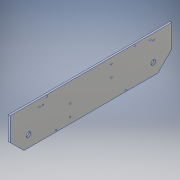
# Autodesk Inventor part: DriveTrain3.0
Saved by Autodesk Inventor 2019 (Build 230136000, 136)
## iProperties
Created: 2017-07-22
Part Number: DriveTrain3.0
Material: Aluminum 6061
Document SubType Name: Modeling
Designer: User
Density: 2.7 g/cm^3
Appearance: Aluminum - Flat
Mass: 590.045 g
Surface Area: 982.684 cm^2
Volume: 218.535 cm^3
Author: User
Autodesk Inventor part; units mm, degrees
ref_plane "YZ Plane" through (0, 0, 0) normal (1, 0, 0) x (0, 1, 0)
ref_plane "XZ Plane" through (0, 0, 0) normal (0, 1, 0) x (-1, 0, 0)
ref_plane "XY Plane" through (0, 0, 0) normal (0, 0, 1) x (1, 0, 0)
sketch "Sketch1" plane through (0, 0, 0) normal (1, 0, 0) x (0, 1, 0)
  line L0 (0, 0) -> (101.6, 0)
  line L1 (101.6, 0) -> (101.6, -444.5)
  line L2 (101.6, -444.5) -> (0, -444.5)
  line L3 (0, -444.5) -> (0, 0)
  circle A0 centre (31.75, -50.8) radius 6.3627
  circle A1 centre (31.75, -393.7) radius 6.3627
  circle A2 centre (86.2838, -165.5318) radius 1.5875
  circle A3 centre (70.2818, -165.5318) radius 1.5875
  circle A4 centre (15.3162, -278.9682) radius 1.5875
  circle A5 centre (31.3182, -278.9682) radius 1.5875
  dimension "d0" = 101.6
  dimension "d1" = 444.5
  dimension "d2" = 12.7254
  dimension "d3" = 31.75
  dimension "d4" = 50.8
  dimension "d5" = 50.8
  dimension "d22" = 165.5318
  dimension "d23" = 3.175
  dimension "d24" = 15.3162
  dimension "d25" = 3.175
  dimension "d26" = 16.002
  dimension "d27" = 165.5318
  dimension "d28" = 3.175
  dimension "d29" = 15.3162
  dimension "d30" = 165.5318
  dimension "d31" = 3.175
  dimension "d32" = 16.002
  dimension "d33" = 165.5318
  constraints: 8 end point, 6 centre point, 2 parallel, 1 horizontal, 1 perpendicular
  measures "d0" distance of L1.end L2.end
  measures "d1" distance of L0.end L1.end
  measures "d2" diameter of A0
  measures "d3" distance from line of L3 A0.centre
  measures "d4" distance from line of L0 A0.centre
  measures "d5" distance from line of L2 A1.centre
  measures "d22" distance from line of L0 A2.centre
  measures "d23" diameter of A2
  measures "d24" distance from line of L1 A2.centre
  measures "d25" diameter of A3
  measures "d26" distance of A2.centre A3.centre
  measures "d27" distance from line of L0 A3.centre
  measures "d28" diameter of A4
  measures "d29" distance from line of L3 A4.centre
  measures "d30" distance from line of L2 A4.centre
  measures "d31" diameter of A5
  measures "d32" distance of A5.centre A4.centre
  measures "d33" distance from line of L2 A5.centre
extrude "Extrusion1" add sketch "Sketch1" along normal blind 4.7625 contours L0 L1 L2 L3 | A2 | A3 | A4 | A5
chamfer "Chamfer1" distance 38.1 angle 45 1 edges at (2.3813, 0, 0)
chamfer "Chamfer2" distance 38.1 angle 45 1 edges at (2.3813, 0, -444.5)
sketch "Sketch6" plane through (4.7625, 0, 0) normal (1, 0, 0) x (0, 0, -1)
  line L0 (444.5, 38.1) -> (406.4, 0) projected
  line L1 (444.5, 38.1) -> (444.5, 101.6) projected
  line L2 (444.5, 101.6) -> (0, 101.6) projected
  line L3 (0, 101.6) -> (0, 38.1) projected
  line L4 (38.1, 0) -> (0, 38.1) projected
  line L5 (38.1, 0) -> (406.4, 0) projected
  circle A0 centre (393.7, 31.75) radius 6.3627 projected
  circle A1 centre (50.8, 31.75) radius 6.3627 projected
  point P0 (0, 0)
  point P1 (165.7604, 16.002)
  point P2 (165.7604, 48.006)
  point P3 (278.7396, 85.598)
  point P4 (278.7396, 53.594)
  dimension "d82" = 32.004
  dimension "d83" = 16.002
  dimension "d84" = 32.004
  dimension "d85" = 16.002
  measures "d82" distance of point (165.76, 16.002) point (165.76, 48.006)
  measures "d83" distance from line of L5 point (165.76, 16.002)
  measures "d84" distance of point (278.74, 53.594) point (278.74, 85.598)
  measures "d85" distance from line of L2 point (278.74, 85.598)
hole "Hole1" at (4.7625, 16.002, -165.7604) at (4.7625, 48.006, -165.7604) at (4.7625, 85.598, -278.7396) at (4.7625, 53.594, -278.7396) direction (-1, 0, 0) diameter 3.81 end through all
sketch "Sketch7" plane through (4.7625, 0, 0) normal (1, 0, 0) x (0, 0, -1)
  circle A0 centre (278.7396, 85.598) radius 1.905 projected
  circle A1 centre (165.7604, 16.002) radius 1.905 projected
  circle A2 centre (165.7604, 48.006) radius 1.905 projected
  circle A3 centre (278.7396, 53.594) radius 1.905 projected
  line L0 (444.5, 38.1) -> (406.4, 0) projected
  line L1 (444.5, 38.1) -> (444.5, 101.6) projected
  line L2 (444.5, 101.6) -> (0, 101.6) projected
  line L3 (0, 101.6) -> (0, 38.1) projected
  line L4 (38.1, 0) -> (0, 38.1) projected
  line L5 (38.1, 0) -> (406.4, 0) projected
  circle A4 centre (393.7, 31.75) radius 6.3627 projected
  circle A5 centre (50.8, 31.75) radius 6.3627 projected
  line L6 (394.4901, 84.4283) -> (386.08, 88.9)
  circle A6 centre (386.08, 88.9) radius 9.525
  point P0 (0, 0)
  point P1 (80.9625, 82.55)
  point P2 (90.4875, 82.55)
  dimension "d102" = 19.05
  dimension "d95" = 19.05
  dimension "d96" = 19.05
  dimension "d97" = 9.525
  dimension "d98" = 80.9625
  dimension "d99" = 12.7
  dimension "d100" = 58.42
  dimension "d101" = 28
  constraints: 2 end point, 1 coincident, 3 other
  measures "d95" distance from line of L2 point (90.487, 82.55)
  measures "d96" distance from line of L2 point (80.962, 82.55)
  measures "d97" distance of point (90.487, 82.55) point (80.962, 82.55)
  measures "d98" distance from line of L3 point (80.962, 82.55)
  measures "d99" distance from line of L2 L6.end
  measures "d100" distance from line of L1 L6.end
  measures "d101" angle of L2 L6
hole "Hole2" at (4.7625, 82.55, -80.9625) at (4.7625, 82.55, -90.4875) at (4.7625, 88.9, -386.08) at (4.7625, 84.4283, -394.4901) direction (-1, 0, 0) diameter 3.81 depth 25.4 tip angle 118
sketch "Sketch8" plane through (4.7625, 0, 0) normal (1, 0, 0) x (0, 0, -1)
  circle A0 centre (386.08, 88.9) radius 1.905 projected
  circle A1 centre (80.9625, 82.55) radius 1.905 projected
  circle A2 centre (90.4875, 82.55) radius 1.905 projected
  circle A3 centre (394.4901, 84.4283) radius 1.905 projected
  circle A4 centre (278.7396, 85.598) radius 1.905 projected
  circle A5 centre (165.7604, 16.002) radius 1.905 projected
  circle A6 centre (165.7604, 48.006) radius 1.905 projected
  circle A7 centre (278.7396, 53.594) radius 1.905 projected
  line L0 (444.5, 38.1) -> (406.4, 0) projected
  line L1 (444.5, 38.1) -> (444.5, 101.6) projected
  line L2 (444.5, 101.6) -> (0, 101.6) projected
  line L3 (0, 101.6) -> (0, 38.1) projected
  line L4 (38.1, 0) -> (0, 38.1) projected
  line L5 (38.1, 0) -> (406.4, 0) projected
  circle A8 centre (393.7, 31.75) radius 6.3627 projected
  circle A9 centre (50.8, 31.75) radius 6.3627 projected
  point P0 (0, 0)
  point P1 (101.6, 97.155)
  point P2 (342.9, 97.155)
  point P3 (127, 4.445)
  point P4 (317.5, 4.445)
  dimension "d110" = 4.445
  dimension "d111" = 4.445
  dimension "d112" = 101.6
  dimension "d113" = 101.6
  dimension "d114" = 4.445
  dimension "d115" = 4.445
  dimension "d123" = 127
  dimension "d124" = 127
  measures "d110" distance from line of L2 point (342.9, 97.155)
  measures "d111" distance from line of L2 point (101.6, 97.155)
  measures "d112" distance from line of L3 point (101.6, 97.155)
  measures "d113" distance from line of L1 point (342.9, 97.155)
  measures "d114" distance from line of L5 point (317.5, 4.445)
  measures "d115" distance from line of L5 point (127, 4.445)
  measures "d123" distance from line of L1 point (317.5, 4.445)
  measures "d124" distance from line of L3 point (127, 4.445)
hole "Hole3" at (4.7625, 97.155, -101.6) at (4.7625, 97.155, -342.9) at (4.7625, 4.445, -127) at (4.7625, 4.445, -317.5) direction (-1, 0, 0) diameter 3.81 depth 25.4 tip angle 118
equation "\"d96\" = d95"
equation "\"d110\" = d111"
equation "\"d112\" = d113"
equation "\"d114\" = d111"
equation "\"d115\" = d111"
equation "\"d124\" = d123"
body "Solid1"
